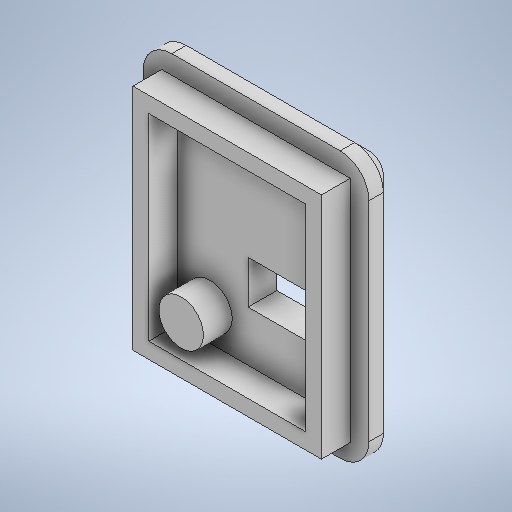
# Autodesk Inventor part: VL53L0X_cover
Saved by Autodesk Inventor 2025.3 (Build 293356000, 356)
## iProperties
Created: 2025-11-14
Part Number: VL53L0X_cover
Material: Generic
Document SubType Name: Modeling
Designer: woyao
Density: 1 g/cm^3
Appearance: Default
Author: woyao
Autodesk Inventor part; units mm, degrees
ref_plane "YZ Plane" through (0, 0, 0) normal (1, 0, 0) x (0, 1, 0)
ref_plane "XZ Plane" through (0, 0, 0) normal (0, 1, 0) x (-1, 0, 0)
ref_plane "XY Plane" through (0, 0, 0) normal (0, 0, 1) x (1, 0, 0)
sketch "Sketch1" plane through (0, 0, 0) normal (0, 0, 1) x (1, 0, 0)
  point P0 (0, 0)
sketch "Sketch2" plane through (0, 0, 0) normal (0, 0, 1) x (1, 0, 0)
  point P0 (0, 0)
sketch "Sketch3" plane through (0, 0, 0) normal (0, 0, 1) x (1, 0, 0)
  line L0 (0, 0) -> (10.9, 0)
  line L1 (10.9, 0) -> (10.9, 13.7)
  line L2 (10.9, 13.7) -> (0, 13.7)
  line L3 (0, 13.7) -> (0, 0)
  line L4 (-1.1, -1.1) -> (12, -1.1)
  line L5 (12, -1.1) -> (12, 14.8)
  line L6 (12, 14.8) -> (-1.1, 14.8)
  line L7 (-1.1, 14.8) -> (-1.1, -1.1)
  dimension "d0" = 13.7
  dimension "d1" = 10.9
  dimension "d7" = 1.1
  constraints: 16 end point, 4 parallel, 2 perpendicular, 1 horizontal, 3 other
  measures "d0" distance of L2.end L0.start
  measures "d1" distance of L0.start L0.end
  measures "d7" distance between parallel lines of L3 L7
extrude "Extrusion1" add sketch "Sketch3" along normal blind 2
sketch "Sketch5" plane through (0, 0, 0) normal (0, 0, -1) x (-1, 0, 0)
  line L0 (-12, 14.8) -> (1.1, 14.8) projected
  line L1 (-12, -1.1) -> (-12, 14.8) projected
  line L2 (1.1, 14.8) -> (1.1, -1.1) projected
  line L3 (1.1, -1.1) -> (-12, -1.1) projected
  line L4 (2.4, 16.1) -> (-13.3, 16.1)
  line L5 (-13.3, 16.1) -> (-13.3, -2.4)
  line L6 (-13.3, -2.4) -> (2.4, -2.4)
  line L7 (2.4, -2.4) -> (2.4, 16.1)
  point P0 (0, 0)
  dimension "d8" = 1.3
  constraints: 8 end point, 3 other
  measures "d8" distance between parallel lines of L0 L4
extrude "Extrusion2" add sketch "Sketch5" along normal blind 2 contours L0 L2 L3 L1 | L7 L6 L5 L4
sketch "Sketch6" plane through (0, 0, 0) normal (0, 0, 1) x (1, 0, 0)
  circle A0 centre (2.25, 2.25) radius 1.55
  line L0 (0, 0) -> (0, 13.7) projected
  line L1 (10.9, 0) -> (0, 0) projected
  dimension "d11" = 3.1
  dimension "d12" = 2.25
  dimension "d13" = 2.25
  constraints: 1 centre point
  measures "d11" diameter of A0
  measures "d12" distance from line of L0 A0.centre
  measures "d13" distance from line of L1 A0.centre
extrude "Extrusion3" add sketch "Sketch6" along normal blind 2
sketch "Sketch7" plane through (0, 0, 0) normal (0, 0, 1) x (1, 0, 0)
  line L0 (4.9, 3.5) -> (10.9, 3.5)
  line L1 (10.9, 3.5) -> (10.9, 6.5)
  line L2 (10.9, 6.5) -> (4.9, 6.5)
  line L3 (4.9, 6.5) -> (4.9, 3.5)
  line L4 (0, 0) -> (0, 13.7) projected
  line L5 (10.9, 0) -> (0, 0) projected
  line L6 (10.9, 13.7) -> (10.9, 0) projected
  dimension "d16" = 3
  dimension "d17" = 6
  dimension "d22" = 3.5
  dimension "d23" = 0
  constraints: 8 end point, 2 parallel, 1 horizontal, 1 perpendicular
  measures "d16" distance of L2.end L0.start
  measures "d17" distance of L0.start L0.end
  measures "d22" distance between parallel lines of L5 L0
  measures "d23" distance between parallel lines of L6 L1
extrude "Extrusion4" cut sketch "Sketch7" against normal blind 2
fillet "Fillet1" radius 2 4 edges at (13.3, 16.1, -1) (-2.4, 16.1, -1) (13.3, -2.4, -1) (-2.4, -2.4, -1)
chamfer "Chamfer1" distance 1 angle 45 8 edges at (5.45, 16.1, -2) (12.7142, 15.5142, -2) (13.3, 6.85, -2) (12.7142, -1.8142, -2) (5.45, -2.4, -2) (-1.8142, -1.8142, -2) (-2.4, 6.85, -2) (-1.8142, 15.5142, -2)
equation "\"d13\" = d12"
body "Solid1"
